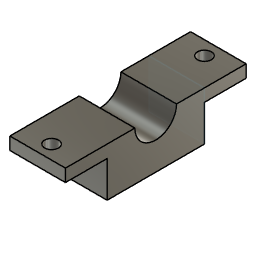
SOPORTE v1 (Autodesk Fusion 360 design; units mm, degrees)
Autodesk Fusion 360 part; units mm, degrees
sketch "Boceto1" plane through (0, 0, 0) normal (1, 0, 0) x (0, 1, 0)
  line L0 (-30, 20) -> (5, 20)
  line L1 (5, 20) -> (5, -15)
  line L2 (5, -15) -> (-30, -15)
  line L3 (-30, -15) -> (-30, 20)
  constraint horizontal L0
  constraint vertical L1
  constraint horizontal L2
  constraint vertical L3
extrude "Extruir1" add sketch "Boceto1" along normal blind 20
sketch "Boceto2" plane through (20, 0, 0) normal (1, 0, 0) x (0, 1, 0)
  line L0 (-30, -15) -> (5, -15)
  line L1 (5, -15) -> (5, 20)
  line L2 (5, 20) -> (-30, 20)
  line L3 (-30, 20) -> (-30, -15)
  circle A0 centre (-12.543, 2.5) radius 7.5
  dimension "d3" = 15
  measures "d3" diameter of A0
extrude "Extruir2" cut sketch "Boceto2" against normal blind 20 contours A0
sketch "Boceto3" plane through (20, 0, 0) normal (1, 0, 0) x (0, 1, 0)
  circle A0 centre (-12.543, 2.5) radius 7.5
  line L0 (-30, -15) -> (5, -15)
  line L1 (5, -15) -> (5, 20)
  line L2 (5, 20) -> (-30, 20)
  line L3 (-30, 20) -> (-30, -15)
  line L4 (-30, 2.5) -> (5, 2.5)
  line L5 (5, 2.5) -> (5, 20)
  line L6 (5, 20) -> (-30, 20)
  line L7 (-30, 20) -> (-30, 2.5)
  constraint horizontal L4
  constraint vertical L5
  constraint horizontal L6
  constraint vertical L7
  constraint coincident L1.end L2.start
  constraint midpoint L3 L4.start
extrude "Extruir3" cut sketch "Boceto3" against normal blind 20 contours A0 L1 L2 L3 L4 L5 L6 L7
sketch "Boceto4" plane through (0, -30, 0) normal (0, -1, 0) x (1, 0, 0)
  line L0 (20, 2.5) -> (0, 2.5)
  line L1 (0, 2.5) -> (0, -15)
  line L2 (0, -15) -> (20, -15)
  line L3 (20, -15) -> (20, 2.5)
  line L4 (0, 2.5) -> (20, 2.5)
  line L5 (20, 2.5) -> (20, -2)
  line L6 (20, -2) -> (0, -2)
  line L7 (0, -2) -> (0, 2.5)
  constraint horizontal L4
  constraint vertical L5
  constraint horizontal L6
  constraint vertical L7
  constraint coincident L3 L5.end
  constraint coincident L0.end L1.start
extrude "Extruir4" add sketch "Boceto4" along normal blind 15 contours L0 L1 L3 L4 L5 L6 L7
sketch "Boceto5" plane through (0, 5, 0) normal (0, 1, 0) x (-1, 0, 0)
  line L0 (0, 2.5) -> (-20, 2.5)
  line L1 (-20, 2.5) -> (-20, -15)
  line L2 (-20, -15) -> (0, -15)
  line L3 (0, -15) -> (0, 2.5)
sketch "Boceto6" plane through (0, 5, 0) normal (0, 1, 0) x (-1, 0, 0)
  line L0 (-20, 2.5) -> (0, 2.5)
  line L1 (0, 2.5) -> (0, -2)
  line L2 (0, -2) -> (-20, -2)
  line L3 (-20, -2) -> (-20, 2.5)
  constraint horizontal L0
  constraint vertical L1
  constraint horizontal L2
  constraint vertical L3
extrude "Extruir5" add sketch "Boceto6" along normal blind 15
sketch "Boceto7" plane through (0, 0, 2.5) normal (0, 0, 1) x (-1, 0, 0)
  line L0 (-20, 45) -> (-20, 20.043)
  line L1 (-20, 20.043) -> (0, 20.043)
  line L2 (0, 20.043) -> (0, 45)
  line L3 (0, 45) -> (-20, 45)
  circle A0 centre (-10, 40) radius 2.5
  circle A1 centre (-10, -15) radius 2.5
  dimension "d12" = 5
  dimension "d13" = 5
  measures "d12" diameter of A0
  measures "d13" diameter of A1
extrude "Extruir6" cut sketch "Boceto7" against normal blind 4.5 contours A0 | A1
